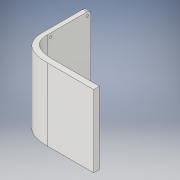
# Autodesk Inventor part: Backplate
Saved by Autodesk Inventor 2019 (Build 230136000, 136)
## iProperties
Created: 2019-04-15
Part Number: Backplate
Material: ABS Plastic
Document SubType Name: Modeling
Designer: Jorian Brusind
Density: 1.06 g/cm^3
Appearance: Smooth - White
Mass: 49.8029 g
Surface Area: 278.333 cm^2
Volume: 46.9839 cm^3
Author: Jorian Brusind
Autodesk Inventor part; units mm, degrees
ref_plane "YZ Plane" through (0, 0, 0) normal (1, 0, 0) x (0, 1, 0)
ref_plane "XZ Plane" through (0, 0, 0) normal (0, 1, 0) x (-1, 0, 0)
ref_plane "XY Plane" through (0, 0, 0) normal (0, 0, 1) x (1, 0, 0)
sketch "Sketch1" plane through (0, 0, 0) normal (0, 1, 0) x (-1, 0, 0)
  line L0 (0, 0) -> (63, 0)
  line L1 (0, 0) -> (0, -5)
  line L2 (0, -5) -> (63, -5)
  line L3 (0, -5) -> (0, -50)
  line L4 (0, -50) -> (100, -50)
  line L5 (100, -50) -> (97, -50)
  line L6 (97, -50) -> (97, -30)
  line L7 (63, -5) -> (97, -5) construction
  line L8 (97, -5) -> (97, -30) construction
  spline S0 degree 2 poles (63, -5) (97, -5) (97, -30) knots 1 1 1 2 2 2
  line L9 (100, -50) -> (100, -30)
  line L10 (100, -30) -> (100.5429, 0) construction
  line L11 (100.5429, 0) -> (63, 0) construction
  spline S1 degree 2 poles (100, -30) (100.5429, 0) (63, 0) knots 1 1 1 2 2 2
  line L12 (97, -50) -> (97, -90)
  line L13 (97, -50) -> (137, -50) construction
  line L14 (97, -90) -> (100, -90)
  line L15 (100, -90) -> (100, -50)
  dimension "d0" = 63
  dimension "d1" = 5
  dimension "d2" = 45
  dimension "d3" = 100
  dimension "d4" = 90
  dimension "d5" = 3
  dimension "d6" = 20
  dimension "d7" = 40
  dimension "d8" = 90
  dimension "d9" = 3
  constraints: 24 end point, 5 perpendicular, 5 vertical, 4 horizontal, 1 point on line, 6 other
  measures "d0" distance of L0.start L0.end
  measures "d1" distance of L0.start L1.end
  measures "d2" distance of L1.end L3.end
  measures "d3" distance of L3.end L4.end
  measures "d4" angle of L4 L3
  measures "d5" distance of L4.end L5.end
  measures "d6" distance of L5.end L6.end
  measures "d7" distance of L5.end L12.end
  measures "d8" angle of L12 L13
  measures "d9" distance of L12.end L14.end
extrude "Extrusion1" add sketch "Sketch1" along normal blind 99 contours L0 S1 L9 L4 L6 S0 L2 L1 | L15 L14 L12 L4
fillet "Fillet1" radius 5 2 edges at (-98.5, 0, -90) (-98.5, 99, -90)
sketch "Sketch3" plane through (-100, 0, -30) normal (-1, 0, 0) x (0, 0, 1)
  line L0 (-60, 5) -> (-60, 94) projected
  line L1 (-60, 5) -> (-55, 5)
  line L2 (-55, 0) -> (0, 0) projected
  line L3 (-55, 0) -> (-55, 5)
  circle A0 centre (-55, 5) radius 1.55
  arc A1 (-55, 99) -> (-60, 94) centre (-55, 94) ccw projected
  line L4 (-60, 94) -> (-55, 94)
  line L5 (-55, 94) -> (-55, 99)
  line L6 (0, 0) -> (0, 99) projected
  line L7 (0, 0) -> (0, 5)
  line L8 (0, 5) -> (-5, 5)
  line L9 (0, 99) -> (0, 94)
  line L10 (0, 94) -> (-5, 94)
  circle A2 centre (-5, 5) radius 1.55
  circle A3 centre (-5, 94) radius 1.55
  circle A4 centre (-55, 94) radius 1.55
  point P0 (30, 0)
  dimension "d21" = 5
  dimension "d22" = 5
  dimension "d23" = 3.1
  dimension "d24" = 5
  dimension "d25" = 5
  dimension "d26" = 5
  dimension "d27" = 5
  dimension "d28" = 3.1
  dimension "d29" = 3.1
  dimension "d30" = 3.1
  constraints: 16 end point, 4 centre point, 4 coincident, 3 perpendicular, 2 horizontal, 2 point on line, 1 vertical
  measures "d21" distance of L0.start L1.end
  measures "d22" distance of L2.start L3.end
  measures "d23" diameter of A0
  measures "d24" distance of L2.end L7.end
  measures "d25" distance of L7.end L8.end
  measures "d26" distance of L6.end L9.end
  measures "d27" distance of L9.end L10.end
  measures "d28" diameter of A2
  measures "d29" diameter of A3
  measures "d30" diameter of A4
extrude "Extrusion3" cut sketch "Sketch3" against normal blind 3 contours A0 L3 L1 | L1 L3 A0 | A4 L4 L5 | L5 L4 A4 | A2 | A3
thicken "Thicken1" operation add thickness 3 both sides no extend neighbours yes toward (0, 0, 1) faces at (-42, 33, 0) (-67.0539, 49.5, -0.0926) (-100, 63.9081, -51.9602)
body "Solid1"
